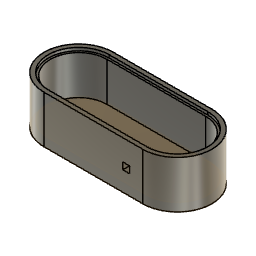
Base (Autodesk Fusion 360 design; units mm, degrees)
Autodesk Fusion 360 part; units mm, degrees
sketch "Sketch1" plane through (0, 0, 0) normal (0, 0, 1) x (1, 0, 0)
  line L0 (0, -33) -> (94, -33)
  arc A0 (94, -33) -> (94, 33) centre (94, 0) ccw
  line L1 (94, 33) -> (0, 33)
  arc A1 (0, 33) -> (0, -33) centre (0, 0) ccw
  line L2 (0, 0) -> (94, 0) construction
  point P0 (-33, 0)
  point P1 (127, 0)
  dimension "d1" = 94
  dimension "d2" = 66
  dimension "d3" = 33
  dimension "d4" = 160
  constraint tangent L0 A0
  constraint tangent A0 L1
  constraint parallel L0 L1
  constraint tangent L1 A1
  constraint tangent L0 A1
  constraint horizontal L2
  constraint coincident A1.centre L2.start
  constraint midpoint A1 P0
  constraint midpoint A0 P1
  measures "d1" distance of A1.centre A0.centre
  measures "d2" diameter of A0
  measures "d3" distance of A1.centre P0
  measures "d4" distance of P0 P1
extrude "Extrude1" add sketch "Sketch1" along normal blind 40
move_face "OffsetFaces1" offset 5 1 faces at (62.6667, -11, 40)
sketch "Sketch2" plane through (0, 0, 45) normal (0, 0, 1) x (-1, 0, 0)
  arc A0 (0, -33) -> (0, 33) centre (0, 0) ccw
  line L0 (0, 33) -> (-94, 33)
  arc A1 (-94, 33) -> (-94, -33) centre (-94, 0) ccw
  line L1 (-94, -33) -> (0, -33)
  line L2 (0, 29) -> (-94, 29)
  arc A2 (-94, 29) -> (-94, -29) centre (-94, 0) ccw
  line L3 (-94, -29) -> (0, -29)
  arc A3 (0, -29) -> (0, 29) centre (0, 0) ccw
  dimension "d8" = -4
extrude "Extrude2" cut sketch "Sketch2" against normal blind 40 contours L2 A2 L3 A3
sketch "Sketch3" plane through (0, 0, 5) normal (0, 0, 1) x (-1, 0, 0)
  arc A0 (0, -29) -> (0, 29) centre (0, 0) ccw
  line L0 (0, 29) -> (-94, 29)
  arc A1 (-94, 29) -> (-94, -29) centre (-94, 0) ccw
  line L1 (-94, -29) -> (0, -29)
  line L2 (0, 27) -> (-94, 27)
  arc A2 (-94, 27) -> (-94, -27) centre (-94, 0) ccw
  line L3 (-94, -27) -> (0, -27)
  arc A3 (0, -27) -> (0, 27) centre (0, 0) ccw
  dimension "d11" = -2
sketch "Sketch4" plane through (0, 0, 5) normal (0, 0, 1) x (-1, 0, 0)
  arc A0 (0, -29) -> (0, 29) centre (0, 0) ccw
  line L0 (0, 29) -> (-94, 29)
  arc A1 (-94, 29) -> (-94, -29) centre (-94, 0) ccw
  line L1 (-94, -29) -> (0, -29)
extrude "Extrude3" add sketch "Sketch3" along normal blind 2
move_face "MoveFace1" by (0, 0, 30) 1 faces at (31.3333, 28.3333, 7)
move_face "MoveFace2" by (0, 0, 7.8672) 1 faces at (31.3333, 28.3333, 37)
move_face "MoveFace3" by (0, 0, 0.08) 1 faces at (31.3333, 28.3333, 44.8672)
move_face "MoveFace4" by (0, 0, 0.05) 1 faces at (31.3333, 28.3333, 44.9472)
move_face "MoveFace5" by (0, -5, -2.8) 1 faces at (31.3333, 28.3333, 44.9972)
sketch "Sketch5" plane through (0, 0, 0) normal (0, 0, 1) x (1, 0, 0)
sketch "Sketch6" plane through (0, 0, 0) normal (0, 0, 1) x (1, 0, 0)
  line L0 (-20, 10) -> (35, 10)
  line L1 (35, 10) -> (35, -20)
  line L2 (35, -20) -> (-20, -20)
  line L3 (-20, -20) -> (-20, 10)
  constraint horizontal L0
  constraint vertical L1
  constraint horizontal L2
  constraint vertical L3
sketch "Sketch8" plane through (0, 0, 0) normal (0, 0, -1) x (1, 0, 0)
  arc A0 (0, 33) -> (0, -33) centre (0, 0) ccw
  line L0 (0, -33) -> (94, -33)
  arc A1 (94, -33) -> (94, 33) centre (94, 0) ccw
  line L1 (94, 33) -> (0, 33)
sketch "Sketch9" plane through (0, -33, 0) normal (0, -1, 0) x (1, 0, 0)
  line L0 (0, 0) -> (94, 0)
  line L1 (94, 0) -> (94, 45)
  line L2 (94, 45) -> (0, 45)
  line L3 (0, 45) -> (0, 0)
  line L4 (75, 25) -> (81.5, 25)
  line L5 (81.5, 25) -> (81.5, 18.5)
  line L6 (81.5, 18.5) -> (75, 18.5)
  line L7 (75, 18.5) -> (75, 25)
  dimension "d22" = 6.5
  dimension "d23" = 6.5
  constraint horizontal L4
  constraint vertical L5
  constraint horizontal L6
  constraint vertical L7
  measures "d22" distance of L4.start L4.end
  measures "d23" distance of L4.start L6.end
extrude "Extrude7" cut sketch "Sketch9" against normal blind 15 contours L4 L5 L6 L7
